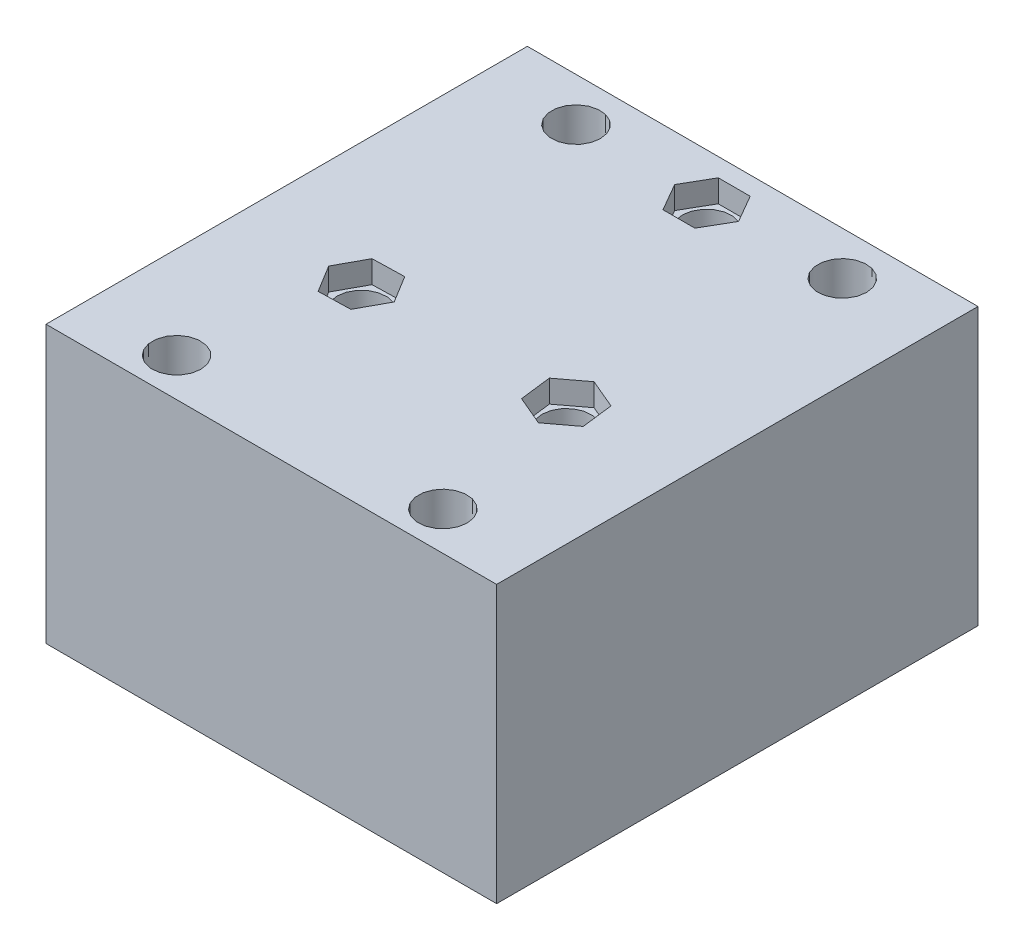
# Autodesk Inventor part: adapter-optical
Saved by Autodesk Inventor 2026.2 (Build 302298000, 298)
## iProperties
Created: 2026-05-22
Part Number: adapter-optical
Material: Generic
Document SubType Name: Modeling
Designer: mayhe
Density: 1 g/cm^3
Appearance: Default
Author: mayhe
Autodesk Inventor part; units mm, degrees
ref_plane "YZ Plane" through (0, 0, 0) normal (1, 0, 0) x (0, 1, 0)
ref_plane "XZ Plane" through (0, 0, 0) normal (0, 1, 0) x (-1, 0, 0)
ref_plane "XY Plane" through (0, 0, 0) normal (0, 0, 1) x (1, 0, 0)
sketch "Sketch1" plane through (0, 0, 0) normal (1, 0, 0) x (0, 1, 0)
  line L0 (13.5, 23.5) -> (-13.5, 23.5)
  line L1 (-13.5, 23.5) -> (-13.5, -23.5)
  line L2 (-13.5, -23.5) -> (13.5, -23.5)
  line L3 (13.5, -23.5) -> (13.5, 23.5)
  line L4 (13.5, 23.5) -> (-13.5, -23.5) construction
  line L5 (-13.5, 23.5) -> (13.5, -23.5) construction
  point P0 (0, 0)
  dimension "d0" = 27
  dimension "d1" = 47
  constraints: 12 end point, 2 midpoint, 2 parallel, 1 horizontal, 1 perpendicular
  measures "d0" distance of L2.end L1.end
  measures "d1" distance of L1.end L0.end
extrude "Extrusion1" add sketch "Sketch1" along normal mid plane 44
sketch "Sketch2" plane through (-22, -13.5, -23.5) normal (0, -1, 0) x (1, 0, 0)
  circle A0 centre (22, 4.5) radius 2.25
  line L0 (0, 0) -> (44, 0) projected
  circle A1 centre (32, 28.2) radius 2.25
  circle A2 centre (12, 28.2) radius 2.25
  point P0 (22, 23.5)
  point P1 (22, 0)
  dimension "d4" = 4.5
  dimension "d5" = 4.5
  dimension "d6" = 4.5
  dimension "d7" = 4.5
  dimension "d8" = 23.7
  dimension "d9" = 10
  dimension "d10" = 10
  constraints: 3 centre point, 1 horizontal alignment, 1 midpoint, 1 vertical alignment
  measures "d4" diameter of A0
  measures "d5" distance from line of L0 A0.centre
  measures "d6" diameter of A1
  measures "d7" diameter of A2
  measures "d8" vertical distance of A1.centre A0.centre
  measures "d9" horizontal distance of A0.centre A1.centre
  measures "d10" horizontal distance of A2.centre A0.centre
hole "Hole1" at (0, -13.5, -19) at (-10, -13.5, 4.7) at (10, -13.5, 4.7) direction (0, 1, 0) diameter 4.75 depth 27 tip angle 118
sketch "Sketch3" plane through (-22, 13.5, 23.5) normal (0, 1, 0) x (1, 0, 0)
  circle A0 centre (22, 42.5) radius 2.375 projected
  circle A1 centre (32, 18.8) radius 2.375 projected
  circle A2 centre (12, 18.8) radius 2.375 projected
  circle A3 centre (22, 42.5) radius 2.7
  circle A4 centre (12, 18.8) radius 2.7
  circle A5 centre (32, 18.8) radius 2.7
  line L0 (20.4412, 39.8) -> (18.8823, 42.5)
  line L1 (18.8823, 42.5) -> (20.4412, 45.2)
  line L2 (20.4412, 45.2) -> (23.5588, 45.2)
  line L3 (23.5588, 45.2) -> (25.1177, 42.5)
  line L4 (25.1177, 42.5) -> (23.5588, 39.8)
  line L5 (23.5588, 39.8) -> (20.4412, 39.8)
  line L6 (10.5097, 16.0616) -> (8.8833, 18.7214)
  line L7 (8.8833, 18.7214) -> (10.3736, 21.4599)
  line L8 (10.3736, 21.4599) -> (13.4903, 21.5384)
  line L9 (13.4903, 21.5384) -> (15.1167, 18.8786)
  line L10 (15.1167, 18.8786) -> (13.6264, 16.1401)
  line L11 (13.6264, 16.1401) -> (10.5097, 16.0616)
  line L12 (32.3812, 15.7057) -> (29.5109, 16.9227)
  line L13 (29.5109, 16.9227) -> (29.1296, 20.017)
  line L14 (29.1296, 20.017) -> (31.6188, 21.8943)
  line L15 (31.6188, 21.8943) -> (34.4891, 20.6773)
  line L16 (34.4891, 20.6773) -> (34.8704, 17.583)
  line L17 (34.8704, 17.583) -> (32.3812, 15.7057)
  point P0 (22, 23.5)
  point P1 (22, 39.8)
  point P2 (12.068, 16.1009)
  point P3 (33.6258, 16.6444)
  dimension "d18" = 5.4
  dimension "d19" = 5.4
  dimension "d20" = 5.4
  constraints: 36 end point, 6 coincident, 3 midpoint, 1 point on line, 1 vertical alignment, 47 other
extrude "Extrusion2" cut sketch "Sketch3" against normal blind 2.2 contours A0 | A1 | A2 | A3 | A3 L3 L4 | A3 L2 L3 | L4 L5 A3 | A3 L1 L2 | L5 L0 A3 | A3 L0 L1 | A4 | A4 L9 L10 | A4 L8 L9 | L10 L11 A4 | A4 L7 L8 | L11 L6 A4 | A4 L6 L7 | A5 | A5 L16 L17 | A5 L15 L16 | L17 L12 A5 | A5 L14 L15 | L12 L13 A5 | A5 L13 L14
sketch "Sketch4" plane through (-22, -13.5, 23.5) normal (0, 1, 0) x (1, 0, 0)
  circle A0 centre (9, 42.75) radius 2.375
  line L0 (0, 47) -> (44, 47) projected
  line L1 (0, 0) -> (0, 47) projected
  circle A1 centre (35, 42.75) radius 2.375
  circle A2 centre (9, 3.75) radius 2.375
  circle A3 centre (35, 3.75) radius 2.375
  point P0 (22, 23.5)
  dimension "d23" = 4.75
  dimension "d24" = 4.25
  dimension "d25" = 9
  dimension "d28" = 26
  dimension "d31" = 39
  constraints: 4 centre point, 1 horizontal, 1 vertical, 6 other
  measures "d23" diameter of A0
  measures "d24" distance from line of L0 A0.centre
  measures "d25" distance from line of L1 A0.centre
  measures "d28" distance of A0.centre A1.centre
  measures "d31" distance of A0.centre A2.centre
hole "Hole2" at (13, -13.5, -19.25) at (-13, -13.5, -19.25) at (-13, -13.5, 19.75) at (13, -13.5, 19.75) direction (0, 1, 0) diameter 4.75 depth 27 tip angle 118 counterbore diameter 5.4 counterbore depth 2
body "Solid1"
